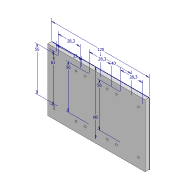
# Autodesk Inventor part: MotorDriverFixation
Saved by Autodesk Inventor 2022 (Build 260153000, 153)
## iProperties
Created: 2022-12-21
Part Number: MotorDriverFixation
Material: Generisch
Document SubType Name: Modeling
Designer: alexw
Density: 1 g/cm^3
Appearance: Vorgabe
Author: alexw
Autodesk Inventor part; units mm, degrees
ref_plane "YZ Plane" through (0, 0, 0) normal (1, 0, 0) x (0, 1, 0)
ref_plane "XZ Plane" through (0, 0, 0) normal (0, 1, 0) x (-1, 0, 0)
ref_plane "XY Plane" through (0, 0, 0) normal (0, 0, 1) x (1, 0, 0)
sketch "Skizze1" plane through (0, 0, 0) normal (0, 0, 1) x (1, 0, 0)
  line L0 (0, 0) -> (125, 0)
  line L1 (125, 0) -> (125, 80)
  line L2 (125, 80) -> (0, 80)
  line L3 (0, 80) -> (0, 0)
  line L4 (6, 70.5) -> (39, 70.5) construction
  line L5 (39, 70.5) -> (39, 9.5) construction
  line L6 (39, 9.5) -> (6, 9.5) construction
  line L7 (6, 9.5) -> (6, 70.5) construction
  line L8 (46, 70.5) -> (79, 70.5) construction
  line L9 (79, 70.5) -> (79, 9.5) construction
  line L10 (79, 9.5) -> (46, 9.5) construction
  line L11 (46, 9.5) -> (46, 70.5) construction
  line L12 (86, 70.5) -> (119, 70.5) construction
  line L13 (119, 70.5) -> (119, 9.5) construction
  line L14 (119, 9.5) -> (86, 9.5) construction
  line L15 (86, 9.5) -> (86, 70.5) construction
  line L16 (6, 40) -> (119, 40) construction
  line L17 (62.5, 70.5) -> (62.5, 9.5) construction
  line L18 (22.5, 70.5) -> (22.5, 9.5) construction
  line L19 (102.5, 70.5) -> (102.5, 9.5) construction
  line L20 (8.35, 68) -> (36.65, 68) construction
  line L21 (8.35, 68) -> (8.35, 12) construction
  line L22 (8.35, 12) -> (36.65, 12) construction
  line L23 (36.65, 12) -> (36.65, 68) construction
  line L24 (62.5, 80) -> (62.5, 0) construction
  line L25 (48.35, 68) -> (76.65, 68) construction
  line L26 (48.35, 68) -> (48.35, 12) construction
  line L27 (48.35, 12) -> (76.65, 12) construction
  line L28 (76.65, 12) -> (76.65, 68) construction
  line L29 (48.35, 68) -> (76.65, 12) construction
  line L30 (48.35, 12) -> (76.65, 68) construction
  line L31 (116.65, 12) -> (116.65, 68) construction
  line L32 (88.35, 68) -> (116.65, 68) construction
  line L33 (88.35, 68) -> (88.35, 12) construction
  line L34 (88.35, 12) -> (116.65, 12) construction
  line L35 (88.35, 68) -> (116.65, 12) construction
  line L36 (88.35, 12) -> (116.65, 68) construction
  point P0 (62.5, 40)
  point P1 (22.5, 68)
  point P2 (8.35, 40)
  point P3 (0, 40)
  point P4 (62.5, 68)
  point P5 (48.35, 40)
  point P6 (62.5, 40)
  point P7 (102.5, 68)
  point P8 (88.35, 40)
  point P9 (102.5, 40)
  dimension "d0" = 80
  dimension "d1" = 125
  dimension "d2" = 40
  dimension "d3" = 33
  dimension "d4" = 61
  dimension "d5" = 28.3
  dimension "d6" = 56
  dimension "d7" = 28.3
  dimension "d8" = 56
  dimension "d9" = 28.3
  dimension "d10" = 56
  constraints: 74 end point, 23 midpoint, 11 parallel, 10 horizontal, 7 point on line, 4 perpendicular, 3 collinear, 3 vertical
  measures "d0" distance between parallel lines of L0 L2
  measures "d1" distance between parallel lines of L1 L3
  measures "d2" distance between parallel lines of L19 L17
  measures "d3" distance of L4.start L4.end
  measures "d4" distance of L6.end L4.start
  measures "d5" distance of L20.end L20.start
  measures "d6" distance of L20.start L21.end
  measures "d7" distance of L28.end L25.start
  measures "d8" distance of L25.start L26.end
  measures "d9" distance of L31.end L35.start
  measures "d10" distance of L35.start L34.start
extrude "Extrusion1" add sketch "Skizze1" along normal blind 5
hole "Bohrung1" at (8.35, 68, 0) at (36.65, 68, 0) at (8.35, 12, 0) at (36.65, 12, 0) at (76.65, 12, 0) at (76.65, 68, 0) at (48.35, 68, 0) at (48.35, 12, 0) at (116.65, 12, 0) at (116.65, 68, 0) at (88.35, 12, 0) at (88.35, 68, 0) direction (0, 0, 1) diameter 2 end through all
